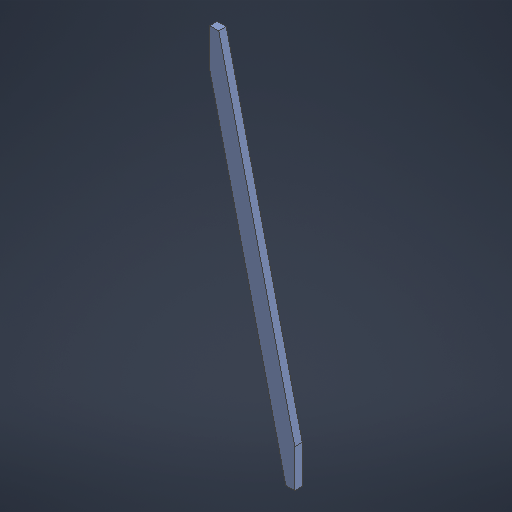
# Autodesk Inventor part: fside1
Saved by Autodesk Inventor 2026 (Build 300175000, 175)
## iProperties
Created: 2024-09-16
Part Number: fside1
Material: Generic
Document SubType Name: Modeling
Designer: User
Density: 1 g/cm^3
Appearance: Default
Author: User
Autodesk Inventor part; units mm, degrees
ref_plane "YZ Plane" through (0, 0, 0) normal (1, 0, 0) x (0, 1, 0)
ref_plane "XZ Plane" through (0, 0, 0) normal (0, 1, 0) x (-1, 0, 0)
ref_plane "XY Plane" through (0, 0, 0) normal (0, 0, 1) x (1, 0, 0)
sketch "Sketch1" plane through (0, 0, 0) normal (0, 0, 1) x (1, 0, 0)
  line L0 (88.9, 914.4) -> (2349.5, 914.4) projected
  line L1 (88.9, -914.4) -> (88.9, 914.4) projected
  line L2 (88.9, -914.4) -> (2349.5, -914.4) projected
  line L3 (520.7, -914.4) -> (520.7, 914.4) projected
  line L4 (2349.5, -914.4) -> (2349.5, 914.4) projected
  line L5 (1917.7, 914.4) -> (1917.7, -914.4) projected
  line L6 (520.7, 743.6248) -> (520.7, -914.4)
  line L7 (88.9, -720.9648) -> (88.9, 914.4)
  line L8 (1917.7, 720.9648) -> (2303.8278, -914.4)
  line L9 (2349.5, -720.9648) -> (1963.3722, 914.4)
  line L10 (88.9, 914.4) -> (520.7, 914.4)
  line L11 (88.9, 914.4) -> (520.7, 914.4)
  line L12 (2303.8278, -914.4) -> (2349.5, -914.4)
  line L13 (2349.5, -720.9648) -> (2349.5, -914.4)
  line L14 (1917.7, 720.9648) -> (1917.7, 914.4)
  line L15 (1917.7, 914.4) -> (1963.3722, 914.4)
  line L16 (520.7, -914.4) -> (88.9, -914.4)
  line L17 (88.9, -914.4) -> (88.9, -720.9648)
  line L18 (88.9, 914.4) -> (520.7, 914.4)
  line L19 (520.7, 738.408) -> (520.7, 914.4)
  line L20 (1917.7, 914.4) -> (2349.5, -914.4)
  line L21 (2306.2395, -924.6143) -> (2392.7605, -904.1857)
  line L22 (1874.4395, 904.1857) -> (1960.9605, 924.6143)
  point P0 (0, 0)
  constraints: 34 end point, 9 point on line, 7 collinear, 2 horizontal, 2 midpoint, 2 parallel, 1 perpendicular, 5 other
extrude "Extrusion1" add sketch "Sketch1" against normal blind 38.1 contours L20 L2 L8 L5 | L0 L9 L4 L20
body "Solid1"
